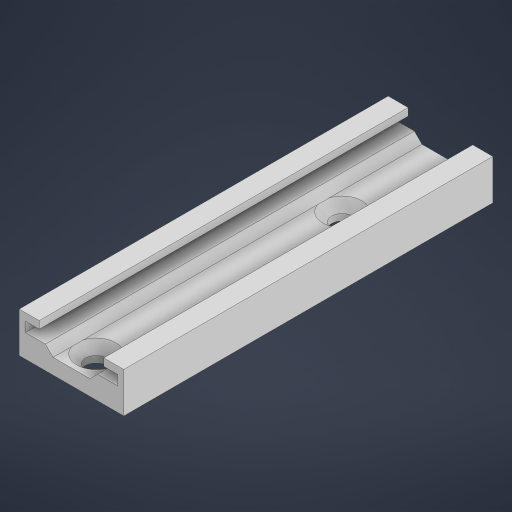
# Autodesk Inventor part: igus_schine
Saved by Autodesk Inventor 2024.2 (Build 282272000, 272)
## iProperties
Created: 2023-12-02
Part Number: igus_schine
Material: Generisch
Document SubType Name: Modeling
Designer: jacob
Density: 1 g/cm^3
Appearance: Vorgabe
Author: jacob
Autodesk Inventor part; units mm, degrees
ref_plane "YZ Plane" through (0, 0, 0) normal (1, 0, 0) x (0, 1, 0)
ref_plane "XZ Plane" through (0, 0, 0) normal (0, 1, 0) x (-1, 0, 0)
ref_plane "XY Plane" through (0, 0, 0) normal (0, 0, 1) x (1, 0, 0)
sketch "Skizze1" plane through (0, 0, 0) normal (0, 0, 1) x (1, 0, 0)
  line L0 (-7.5, 5.35) -> (-5.25, 5.35)
  line L1 (-5.25, 5.35) -> (-5.25, 6.55)
  line L2 (-5.25, 6.55) -> (-8.5, 6.55)
  line L3 (-8.5, 6.55) -> (-8.5, 0)
  line L4 (-8.5, 0) -> (0, 0)
  line L5 (0, 0) -> (0, 2.5)
  line L6 (-4.25, 3.75) -> (-7.5, 3.75)
  line L7 (-7.5, 3.75) -> (-7.5, 5.35)
  line L8 (0, 2.5) -> (-3, 2.5)
  line L9 (-3, 2.5) -> (-4.25, 3.75)
  dimension "d0" = 8.5
  dimension "d1" = 1.6
  dimension "d2" = 7.5
  dimension "d3" = 1.2
  dimension "d4" = 5.25
  dimension "d5" = 6.55
  dimension "d10" = 135
  dimension "d11" = 3
  dimension "d12" = 2.5
  constraints: 20 end point, 6 perpendicular, 2 horizontal, 1 parallel
  measures "d0" distance of L3.end L4.end
  measures "d1" distance of L6.end L0.start
  measures "d2" distance from line of L4.end L7
  measures "d3" distance of L0.end L1.end
  measures "d4" horizontal distance of L5.end L0.end
  measures "d5" distance of L2.end L3.end
  measures "d10" angle of L9 L8
  measures "d11" distance of L5.end L8.end
  measures "d12" distance of L4.end L5.end
extrude "Extrusion1" add sketch "Skizze1" along normal blind 60
mirror "Spiegeln1" about plane through (0, 0, 0) normal (1, 0, 0) of "Extrusion1"
sketch "Skizze2" plane through (-3, 2.5, 60) normal (0, 1, 0) x (1, 0, 0)
  line L0 (3, 72) -> (3, -12) projected
  line L1 (0, 0) -> (6, 0) projected
  point P0 (3, 60)
  point P1 (3, 4)
  point P2 (3, 0)
  point P3 (3, 44)
  dimension "d13" = 4
  dimension "d14" = 40
  constraints: 2 point on line, 1 midpoint
  measures "d13" distance of point (3, 0) point (3, 4)
  measures "d14" distance of point (3, 4) point (3, 44)
hole "Bohrung1" at (0, 2.5, 56) at (0, 2.5, 16) direction (0, -1, 0) diameter 3.4 depth 2.5 countersink diameter 6.3 countersink angle 90 clearance for "Flachkopfmaschinenschraube" size "M3" standard "ANSI Metrisches M Profil"
